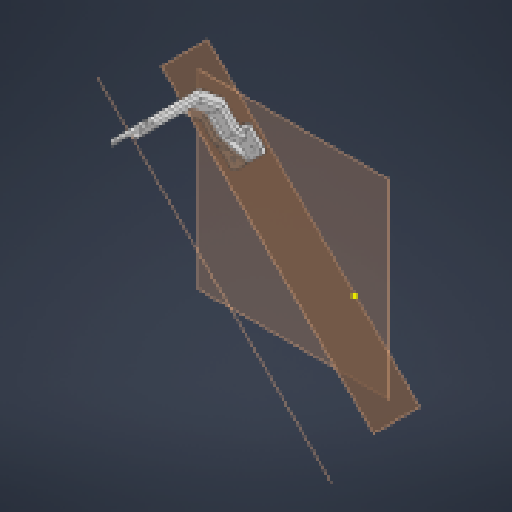
# Autodesk Inventor part: Venstre arm
Saved by Autodesk Inventor 2023.4 (Build 274418000, 418)
## iProperties
Created: 2025-09-26
Part Number: Venstre arm
Material: Generic
Document SubType Name: Modeling
Designer: Malthe Sennels
Density: 1 g/cm^3
Appearance: Default
Author: Malthe Sennels
Autodesk Inventor part; units mm, degrees
ref_plane "YZ Plane" through (0, 0, 0) normal (1, 0, 0) x (0, 1, 0)
ref_plane "XZ Plane" through (0, 0, 0) normal (0, 1, 0) x (-1, 0, 0)
ref_plane "XY Plane" through (0, 0, 0) normal (0, 0, 1) x (1, 0, 0)
ref_plane "Work Plane1" through (0, 0, 0) normal (0, 0, 1) x (1, 0, 0)
sketch "Sketch1" plane through (0, 0, 0) normal (0, 0, 1) x (1, 0, 0)
  line L0 (-14.9261, 58.1475) -> (-18.9164, 56.7911) projected
  arc A0 (-12.4369, -46.9155) -> (-18.9164, 56.7911) centre (-94.7078, 0) ccw projected
  line L1 (-12.4369, -46.9155) -> (-25.0393, -34.3131) projected
  arc A1 (-25.0393, -34.3131) -> (-32.1104, -34.3131) centre (-28.5748, -37.8487) ccw projected
  line L2 (-32.1104, -34.3131) -> (-60.3946, -62.5974) projected
  arc A2 (-60.3946, -62.5974) -> (-60.3946, -69.6685) centre (-56.8591, -66.1329) ccw projected
  line L3 (-60.3946, -69.6685) -> (-47.7922, -82.2709) projected
  arc A3 (-141.6233, -82.2709) -> (-47.7922, -82.2709) centre (-94.7078, 0) ccw projected
  line L4 (-141.6233, -82.2709) -> (-129.0209, -69.6685) projected
  arc A4 (-129.0209, -69.6685) -> (-129.0209, -62.5974) centre (-132.5564, -66.1329) ccw projected
  line L5 (-129.0209, -62.5974) -> (-157.3052, -34.3131) projected
  arc A5 (-157.3052, -34.3131) -> (-164.3762, -34.3131) centre (-160.8407, -37.8487) ccw projected
  line L6 (-164.3762, -34.3131) -> (-176.9786, -46.9155) projected
  arc A6 (-176.9786, 46.9155) -> (-176.9786, -46.9155) centre (-94.7078, 0) ccw projected
  line L7 (-176.9786, 46.9155) -> (-164.3762, 34.3131) projected
  arc A7 (-164.3762, 34.3131) -> (-157.3052, 34.3131) centre (-160.8407, 37.8487) ccw projected
  line L8 (-157.3052, 34.3131) -> (-129.0209, 62.5974) projected
  arc A8 (-129.0209, 62.5974) -> (-129.0209, 69.6685) centre (-132.5564, 66.1329) ccw projected
  line L9 (-129.0209, 69.6685) -> (-141.6233, 82.2709) projected
  arc A9 (-37.9167, 75.7914) -> (-141.6233, 82.2709) centre (-94.7078, 0) ccw projected
  line L10 (-37.9167, 75.7914) -> (-36.5603, 79.7816) projected
  arc A10 (-36.5603, 79.7816) -> (-193.4308, 0) centre (-94.7078, 0) ccw projected
  arc A11 (-193.4308, 0) -> (-94.7078, -98.723) centre (-94.7078, 0) ccw projected
  arc A12 (-94.7078, -98.723) -> (-14.9261, 58.1475) centre (-94.7078, 0) ccw projected
  circle A13 centre (-138.2132, -64.7188) radius 2.25 projected
  circle A14 centre (-159.4265, -43.5055) radius 2.25 projected
  circle A15 centre (-159.4265, 43.5055) radius 2.25 projected
  circle A16 centre (-138.2133, 64.7187) radius 2.25 projected
  circle A17 centre (-51.2022, -64.7187) radius 2.25 projected
  circle A18 centre (-29.989, -43.5055) radius 2.25 projected
  line L11 (-141.6233, 82.2709) -> (-144.5624, 85.21)
  line L12 (-176.9786, 46.9155) -> (-179.9178, 49.8547)
  point P0 (0, 0)
  constraints: 4 end point, 2 point on circle, 1 parallel
extrude "Extrusion1" add sketch "Sketch1" along normal blind 4 contours A10 L11 L9 A8 L8 A7 L7 L12
chamfer "Chamfer1" distance 3 angle 45 1 edges at (-164.5155, 69.8077, 4)
ref_plane "Work Plane2" through (-146.6986, 51.9908, -4) normal (0.7071068, 0.7071068, 0) x (0, 0, 1)
sketch "Sketch2" plane through (-146.6986, 51.9908, -4) normal (0.7071068, 0.7071068, 0) x (0, 0, 1)
  line L0 (8, 0) -> (8, -18.8747) projected
  line L1 (8, -18.8747) -> (8, -22.1969) projected
  line L2 (4, 5) -> (8, 5) projected
  line L3 (8, 5) -> (8, 0)
  line L4 (8, 5) -> (19.8525, -22.7909)
  line L5 (19.8525, -22.7909) -> (19.8525, -46.753)
  line L6 (19.8525, -46.753) -> (29.6486, -56.5491)
  line L7 (29.6486, -56.5491) -> (29.6486, -70.6913)
  line L8 (8, -22.1969) -> (9.8525, -24.0494)
  line L9 (8, -22.1969) -> (10.6198, -22.1969) construction
  line L10 (9.8525, -24.0494) -> (9.8525, -50.8951)
  line L11 (9.8525, -50.8951) -> (29.6486, -70.6913)
  line L12 (25.5065, -66.5491) -> (29.6486, -66.5491)
  point P0 (4, 140.4946)
  dimension "d5" = 135
  dimension "d6" = 45
  dimension "d14" = 10
  dimension "d15" = 10
  dimension "d16" = 10
  constraints: 20 end point, 3 vertical, 2 perpendicular, 2 point on line, 1 equal length, 1 horizontal, 1 parallel
  measures "d5" angle of L6 L5
  measures "d6" angle of L8 L9
  measures "d14" distance from line of L6.end L12
  measures "d15" distance between parallel lines of L5 L10
  measures "d16" distance between parallel lines of L11 L6
extrude "Extrusion2" add sketch "Sketch2" along normal mid plane 6 contours L3 L4 L5 L6 L7 L12 L11 L10 L8 L1 L0
sketch "Sketch3" plane through (-144.5772, 54.1121, -4) normal (0.7071068, 0.7071068, 0) x (-0.7071068, 0.7071068, 0)
  line L0 (22.1969, 8) -> (24.0494, 9.8525) projected
  line L1 (24.0494, 9.8525) -> (50.8951, 9.8525) projected
  line L2 (50.8951, 9.8525) -> (66.5491, 25.5065) projected
  line L3 (56.5491, 29.6486) -> (46.753, 19.8525) projected
  line L4 (46.753, 19.8525) -> (43.753, 16.8525)
  line L5 (43.753, 16.8525) -> (21.1499, 16.8525)
  line L6 (21.1499, 16.8525) -> (12.2974, 8)
  line L7 (22.1499, 8) -> (-5, 8) projected
  line L8 (66.5491, 29.6486) -> (56.5491, 29.6486) projected
  line L9 (22.1499, 8) -> (12.2974, 8)
  line L10 (22.1499, 8) -> (22.1969, 8) projected
  line L11 (66.5491, 25.5065) -> (66.5491, 29.6486) projected
  point P0 (-140.4946, 4)
  point P1 (70.6913, 29.6486)
  dimension "d10" = 7
  dimension "d11" = 7
  constraints: 8 end point, 2 parallel, 1 collinear, 1 horizontal, 1 point on line
  measures "d10" distance between parallel lines of L1 L5
  measures "d11" distance between parallel lines of L6 L0
extrude "Extrusion3" add sketch "Sketch3" along normal blind 15
mirror "Mirror1" about plane through (-146.6986, 51.9908, -4) normal (0.7071068, 0.7071068, 0) of "Extrusion3"
sketch "Sketch4" plane through (-173.9569, 104.705, 25.6486) normal (0, 0, 1) x (0.7071068, 0.7071068, 0)
  point P0 (48.9685, -197.0437)
sketch "Sketch5" plane through (-181.028, 111.7761, 21.5065) normal (-0.7071068, 0.7071068, 0) x (-0.7071068, -0.7071068, 0)
  line L0 (0, 0) -> (0, 4.1421) projected
  line L1 (36, 0) -> (36, 4.1421) projected
  line L2 (36, 4.1421) -> (0, 4.1421) projected
  line L3 (18, 4.1421) -> (18, 69.1421) construction
  circle A0 centre (18, 69.1421) radius 11
  arc A1 (36, 69.1421) -> (0, 69.1421) centre (18, 69.1421) ccw
  line L4 (0, 4.1421) -> (0, 69.1421)
  line L5 (36, 4.1421) -> (36, 69.1421)
  line L6 (18, 51.1421) -> (8, 51.1421)
  line L7 (8, 51.1421) -> (0, 59.1421)
  line L8 (18, 51.1421) -> (28, 51.1421)
  line L9 (28, 51.1421) -> (36, 59.1421)
  point P0 (-48.9685, -21.5065)
  dimension "d17" = 22
  dimension "d18" = 65
  dimension "d21" = 135
  dimension "d22" = 18
  dimension "d23" = 8
  constraints: 14 end point, 2 centre point, 2 coincident, 2 midpoint, 2 point on circle, 2 point on line, 2 symmetric about line, 2 vertical, 1 horizontal, 1 parallel, 1 tangent
  measures "d17" diameter of A0
  measures "d18" distance of point (18, 4.142) L3.end
  measures "d21" angle of L6 L7
  measures "d22" distance from line of L3.end L6
  measures "d23" distance from line of L4 L6.end
extrude "Extrusion4" add sketch "Sketch5" against normal blind 10
chamfer "Chamfer2" distance 3 angle 45 9 edges at (-199.4127, 79.2491, 58.1486) (-186.6848, 91.9771, 108.6486) (-173.9569, 104.705, 58.1486) (-194.8886, 74.725, 19.2505) (-169.4328, 100.1809, 19.2505) (-182.3731, 62.2095, 12.8525) (-156.9173, 87.6654, 12.8525) (-171.2519, 51.0883, 8.4262) (-145.7961, 76.5442, 8.4262)
sketch "Sketch7" plane through (-173.9569, 104.705, 21.5065) normal (0.7071068, -0.7071068, 0) x (0, 0, -1)
  circle A0 centre (-69.1421, -18) radius 11 projected
  line L0 (-69.1421, -18) -> (-10.0348, -18) construction
  line L1 (-51.1421, -18) -> (-51.1421, -30)
  line L2 (-51.1421, -30) -> (-57.1421, -36)
  line L3 (-69.1421, -36) -> (-2.8995, -36) projected
  line L4 (-51.1421, -18) -> (-51.1421, -6)
  line L5 (-51.1421, -6) -> (-57.1421, 0)
  line L6 (-69.1421, -36) -> (-69.1421, -33) projected
  arc A1 (-69.1421, -3) -> (-69.1421, -33) centre (-69.1421, -18) ccw projected
  line L7 (-69.1421, 0) -> (-69.1421, -3) projected
  arc A2 (-69.1421, 0) -> (-69.1421, -36) centre (-69.1421, -18) ccw projected
  line L8 (-2.8995, 0) -> (-69.1421, 0) projected
  point P0 (21.5065, 48.9685)
  dimension "d32" = 135
  dimension "d33" = 6
  dimension "d34" = 18
  constraints: 10 end point, 2 point on line, 2 symmetric about line, 1 horizontal, 1 vertical
  measures "d32" angle of L1 L2
  measures "d33" distance from line of L3 L1.end
  measures "d34" distance of L0.start L1.start
extrude "Extrusion6" cut sketch "Sketch7" against normal blind 5
ref_plane "Work Plane3" through (-146.6986, 51.9908, -4) normal (0.7071068, 0.7071068, 0) x (0, 0, 1)
sketch "Sketch8" plane through (-146.6986, 51.9908, -4) normal (0.7071068, 0.7071068, 0) x (0, 0, 1)
  line L0 (105.6486, -61.5491) -> (83.6486, -61.5491) construction
  line L1 (105.6486, -66.5491) -> (83.6486, -66.5491) projected
  line L2 (105.6486, -61.5491) -> (83.6486, -61.5491) projected
  circle A0 centre (105.4486, -61.5491) radius 2.325
  circle A1 centre (105.4486, -61.5491) radius 2.25 construction
  line L3 (94.6486, -136.2547) -> (94.6486, 225.6844) projected
  point P0 (4, 140.4946)
  dimension "d37" = 4.65
  dimension "d38" = 4.5
  dimension "d39" = 0.2
  constraints: 2 centre point, 1 coincident, 1 point on line
  measures "d37" diameter of A0
  measures "d38" diameter of A1
  measures "d39" distance of L0.start A0.centre
revolve "Revolution1" cut sketch "Sketch8" angle 360 about axis through (-193.7559, 99.0481, 90.6486) along (0.7071068, -0.7071068, 0)
chamfer "Chamfer3" distance 1.5 angle 45 1 edges at (-185.9777, 106.8263, 90.6486)
sketch "Sketch9" plane through (-177.4924, 108.2405, 21.5065) normal (0.7071068, -0.7071068, 0) x (-0.7071068, -0.7071068, 0)
  line L0 (30, -51.1421) -> (36, -57.1421) projected
  line L1 (33, -54.1421) -> (33, -61.2132) construction
  line L2 (33, -54.1421) -> (40.0711, -54.1421) construction
  circle A0 centre (33, -61.2132) radius 1.75
  line L3 (6, -51.1421) -> (30, -51.1421) projected
  line L4 (18, -51.1421) -> (18, -96.5918) construction
  circle A1 centre (3, -61.2132) radius 1.75
  point P0 (-48.9685, 21.5065)
  dimension "d44" = 90
  dimension "d45" = 3.5
  dimension "d46" = 5
  constraints: 6 end point, 2 centre point, 2 coincident, 2 midpoint, 2 symmetric about line, 1 horizontal, 1 perpendicular, 1 vertical, 1 other
  measures "d44" angle of L1 L2
  measures "d45" diameter of A0
  measures "d46" distance from line of L0 L1.end
extrude "Extrusion7" cut sketch "Sketch9" against normal through all
sketch "Sketch10" plane through (-206.4838, 86.3202, 21.5065) normal (-0.7071068, 0.7071068, 0) x (-0.7071068, -0.7071068, 0)
  line L0 (-30.75, 58.9632) -> (-35.25, 58.9632)
  line L1 (-35.25, 58.9632) -> (-35.25, 63.4632)
  line L2 (-35.25, 63.4632) -> (-30.75, 63.4632)
  line L3 (-30.75, 63.4632) -> (-30.75, 58.9632)
  circle A0 centre (-33, 61.2132) radius 1.75 construction
  line L4 (-30.75, 58.9632) -> (-35.25, 63.4632) construction
  line L5 (-35.25, 58.9632) -> (-30.75, 63.4632) construction
  line L6 (-0.75, 58.9632) -> (-5.25, 58.9632)
  line L7 (-5.25, 58.9632) -> (-5.25, 63.4632)
  line L8 (-5.25, 63.4632) -> (-0.75, 63.4632)
  line L9 (-0.75, 63.4632) -> (-0.75, 58.9632)
  circle A1 centre (-3, 61.2132) radius 1.75 construction
  line L10 (-0.75, 58.9632) -> (-5.25, 63.4632) construction
  line L11 (-5.25, 58.9632) -> (-0.75, 63.4632) construction
  point P0 (-84.9685, -21.5065)
  dimension "d49" = 4.5
  dimension "d50" = 4.5
  dimension "d51" = 4.5
  dimension "d52" = 4.5
  constraints: 24 end point, 4 midpoint, 4 parallel, 2 horizontal, 2 perpendicular
  measures "d49" distance of L1.end L2.end
  measures "d50" distance of L0.end L1.end
  measures "d51" distance of L7.end L8.end
  measures "d52" distance of L6.end L7.end
extrude "Extrusion8" cut sketch "Sketch10" against normal blind 3
chamfer "Chamfer4" distance 3 angle 45 3 edges at (-206.4838, 86.3202, 56.0775) (-193.7559, 99.0481, 108.6486) (-181.028, 111.7761, 56.0775)
ref_plane "Work Plane4" through (-146.6986, 51.9908, -4) normal (0.7071068, 0.7071068, 0) x (0, 0, 1)
sketch "Sketch11" plane through (-146.6986, 51.9908, -4) normal (0.7071068, 0.7071068, 0) x (0, 0, 1)
  line L0 (5, -25.1969) -> (8, -22.1969) projected
  line L1 (5, -25.1969) -> (9.8525, -50.8951) construction
  line L2 (9.8525, -24.0494) -> (9.8525, -50.8951) projected
  line L3 (8, -22.1969) -> (9.8525, -24.0494) projected
  line L4 (4.044, -25.5234) -> (10.8525, -61.5805)
  line L5 (10.8525, -61.5805) -> (10.8525, -23.6352)
  line L6 (10.8525, -23.6352) -> (8, -20.7827)
  line L7 (8, -20.7827) -> (4.2929, -24.4898)
  line L8 (9.8525, -50.8951) -> (22.5065, -63.5491) projected
  line L9 (5, -25.1969) -> (4.7754, -24.0074) construction
  arc A0 (9.8525, -50.8951) -> (4.5955, -24.1872) centre (-60.6212, -50.8951) ccw
  point P0 (4, 140.4946)
  point P1 (8, -20.4893)
  point P2 (5, -25.1969)
  point P3 (10.8525, -51.8951)
  dimension "d58" = 1
  constraints: 12 end point, 4 point on circle, 3 point on line, 1 centre point, 1 collinear, 1 tangent, 3 other
  measures "d58" distance between parallel lines of L2 L5
extrude "Extrusion9" add sketch "Sketch11" along normal mid plane 6
body "Solid1"
